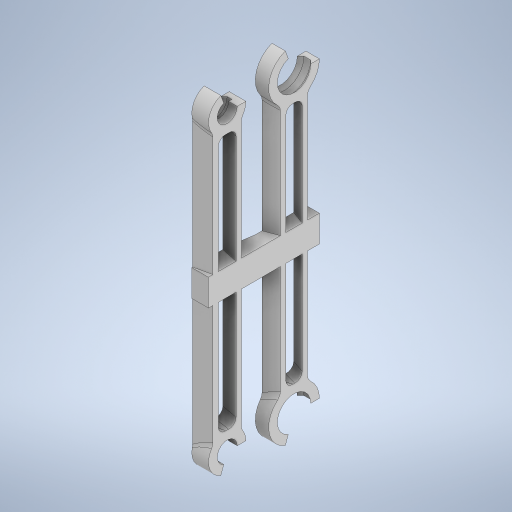
# Autodesk Inventor part: lens mounts
Saved by Autodesk Inventor 2024 (Build 280153000, 153)
## iProperties
Created: 2025-01-15
Part Number: lens mounts
Material: Generic
Document SubType Name: Modeling
Designer: Williamow
Density: 1 g/cm^3
Appearance: Default
Author: Williamow
Autodesk Inventor part; units mm, degrees
ref_plane "YZ Plane" through (0, 0, 0) normal (1, 0, 0) x (0, 1, 0)
ref_plane "XZ Plane" through (0, 0, 0) normal (0, 1, 0) x (-1, 0, 0)
ref_plane "XY Plane" through (0, 0, 0) normal (0, 0, 1) x (1, 0, 0)
sketch "Sketch1" plane through (0, 0, 0) normal (0, 1, 0) x (-1, 0, 0)
  line L0 (2.5, -1.5) -> (2, -2)
  line L1 (2, -2) -> (1.29, -2)
  line L2 (1.29, -2) -> (1.29, -1.5)
  line L3 (1.29, -1.5) -> (0, -1.5)
  line L4 (0, -1.5) -> (0, -2.8)
  line L5 (0, -2.8) -> (2.5, -2.8)
  line L6 (2.5, -2.8) -> (2.5, -1.5)
  line L7 (0, 0) -> (1.5115, 0)
  line L8 (2, -12.5) -> (2, -13.8)
  line L9 (2, -13.8) -> (0, -13.8)
  line L10 (0, -13.8) -> (0, -12.5)
  line L11 (0, -12.5) -> (0.5, -13)
  line L12 (0.5, -13) -> (1.5, -13)
  line L13 (1.5, -13) -> (2, -12.5)
  line L14 (0, -10) -> (1, -10)
  point P0 (1, -13)
  dimension "d0" = 0.5
  dimension "d1" = 45
  dimension "d2" = 0.8
  dimension "d3" = 0.71
  dimension "d4" = 2.5
  dimension "d5" = 2
  dimension "d6" = 1
  dimension "d7" = 0.8
  dimension "d8" = 0.5
  dimension "d9" = 10
  dimension "d10" = 3
  constraints: 30 end point, 8 perpendicular, 3 horizontal, 3 vertical alignment, 2 equal length, 1 horizontal alignment, 1 midpoint, 1 parallel, 1 vertical
  measures "d0" distance of L1.end L2.end
  measures "d1" angle of L6 L0
  measures "d2" distance from line of L5 L1.end
  measures "d3" distance of L0.end L1.end
  measures "d4" distance of L4.end L5.end
  measures "d5" distance between parallel lines of L7 L1
  measures "d6" distance of L11.end L12.end
  measures "d7" distance between parallel lines of L9 L12
  measures "d8" distance from line of L8.start L12
  measures "d9" distance of L14.start L7.start
  measures "d10" distance between parallel lines of L14 L12
revolve "Revolution1" add sketch "Sketch1" angle 250 about axis through (0, 0, 0) along (1, 0, 0) contours L6 L5 L4 L3 L2 L1 L0
revolve "Revolution2" add sketch "Sketch1" angle 250 about axis through (0, 0, -10) along (1, 0, 0) contours L8 L9 L10 L11 L12 L13
ref_plane "Work Plane1" through (-2.5, 20, -2.8) normal (0, -1, 0) x (1, 0, 0)
sketch "Sketch2" plane through (-2.5, 20, -2.8) normal (0, -1, 0) x (1, 0, 0)
  line L0 (0.5, -11) -> (0.5, -3.4) projected
  line L1 (0, 0) -> (0, 5.6) projected
  line L2 (2.5, 0) -> (2.5, 5.6) projected
  line L3 (2.5, -11) -> (2.5, -3.4) projected
  line L4 (2.5, 4.932) -> (0, 5.478)
  line L5 (2.5, 4.122) -> (0, 4.668)
  line L6 (1.25, 5.478) -> (1.25, 4.122) construction
  line L7 (2.5, 2.8) -> (0, 2.8) construction
  line L8 (2.5, 0.668) -> (0, 0.122)
  line L9 (2.5, 1.478) -> (0, 0.932)
  line L10 (2.5, -5.159) -> (0.5, -4.431)
  line L11 (2.5, -5.969) -> (0.5, -5.241)
  line L12 (2.5, -7.2) -> (0.5, -7.2) construction
  line L13 (1.5, -5.969) -> (1.5, -4.431) construction
  line L14 (2.5, -9.241) -> (0.5, -9.969)
  line L15 (2.5, -8.431) -> (0.5, -9.159)
  line L16 (2.5, -11) -> (0.5, -11)
  line L17 (2.5, 0) -> (2.5, -3.4)
  line L18 (0.5, -3.4) -> (0, 0)
  line L19 (2.5, 5.6) -> (0, 5.6)
  point P0 (2.5, 2.8)
  point P1 (0.5, -5.9003)
  point P2 (0, 3.7577)
  point P3 (2.5, 3.7577)
  point P4 (2.5, -5.9003)
  point P5 (1.25, 4.8)
  point P6 (1.25, 4.395)
  point P7 (1.5, -5.2)
  point P8 (1.5, -5.605)
  point P9 (0.5, -9.969)
  point P10 (2.5, -8.431)
  point P11 (0.5, -9.159)
  point P12 (2.5, 1.478)
  point P13 (0, 0.932)
  point P14 (0, 0.122)
  point P15 (2.5, 0.668)
  dimension "d14" = 0.81
  dimension "d16" = 2
  dimension "d18" = 2
  dimension "d19" = 0.81
  dimension "d20" = 70
  dimension "d27" = 1.356
  constraints: 32 end point, 8 midpoint, 8 point on line, 8 symmetric about line, 4 horizontal alignment, 2 parallel, 2 vertical, 2 vertical alignment, 1 collinear, 1 horizontal, 1 perpendicular
  measures "d14" distance of L5.start L4.start
  measures "d16" vertical distance of L7.start point (1.25, 4.8)
  measures "d18" distance from line of L12 point (1.5, -5.2)
  measures "d19" distance of L10.start L11.start
  measures "d20" angle of L3 L11
  measures "d27" distance of L6.start L6.end
extrude "Extrusion1" add sketch "Sketch2" along normal up to next contours L0 L15 L3 L14 | L0 L10 L3 L11 | L1 L9 L2 L8 | L1 L4 L2 L5
extrude "Extrusion2" add sketch "Sketch2" against normal blind 2
fillet "Fillet2" radius 1 8 edges at (-1.3023, 2.2933, 1.6064) (-1.3023, 2.2933, -1.6064) (-1.0247, 3.4449, -8.396) (-1.0247, 3.4449, -11.604) (-1.0517, 2.9266, -12.4238) (-1.4843, 1.3443, -2.4562) (-1.4843, 1.3443, 2.4562) (-1.0517, 2.9266, -7.5762)
mirror "Mirror2" about plane through (-1.25, 22, -5.5) normal (0, 1, 0) of "Extrusion1", "Revolution2", "Revolution1", "Fillet2", "Extrusion2"
body "Solid1"
